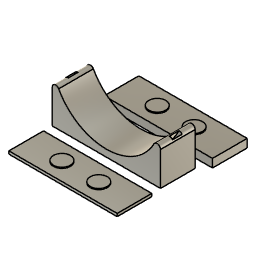
spacer_bandsaw_dust_extraction (Autodesk Fusion 360 design; units mm, degrees)
Autodesk Fusion 360 part; units mm, degrees
sketch "Sketch1" plane through (0, 0, 0) normal (0, 1, 0) x (1, 0, 0)
  circle A0 centre (0, 0) radius 31.25
  line L0 (-31.25, 0) -> (-31.25, 35.25)
  line L1 (-31.25, 35.25) -> (31.25, 35.25)
  line L2 (31.25, 35.25) -> (31.25, 0)
  line L3 (-21.25, 0) -> (-21.25, 33.5)
  line L4 (21.25, 33.5) -> (21.25, 0)
  circle A1 centre (0, 0) radius 32.25
  circle A2 centre (0, 0) radius 34.25
  line L5 (-21.25, 33.5) -> (-21.25, 35.25)
  line L6 (21.25, 33.5) -> (21.25, 35.25)
  dimension "d1" = 62.5
  dimension "d2" = 35.25
  dimension "d3" = 62.5
  dimension "d4" = 10
  dimension "d5" = 10
  dimension "d25" = 1
  dimension "d26" = 3
  constraint coincident A0.centre A1.centre
  constraint coincident A0 L0.start
  constraint tangent A0 L0
  constraint vertical L0
  constraint perpendicular L0 L1
  constraint coincident A0 L2.end
  constraint tangent A0 L2
  constraint coincident L1 L5.end
  constraint perpendicular L1 L5
  constraint coincident L1 L6.end
  constraint perpendicular L1 L6
  measures "d1" diameter of A0
  measures "d2" distance of L0.start L0.end
  measures "d3" distance of L0.end L1.end
extrude "Extrude1" add sketch "Sketch1" along normal blind 20 contours A0 L0 L3 A1 | A0 L2 L4 A1 | A0 L3 L4 A1 | L0 L3 A1 A2 | L2 L4 A1 A2 | L3 L4 A1 A2 | L0 L1 L3 A2 L5 | L1 L2 L4 A2 L6 | L1 L3 L4 A2 L5 L6 makes body 1
fillet "Fillet1" radius 2 2 edges at (-31.25, 10, 0) (31.25, 10, 0) on bodies 1
sketch "Sketch2" plane through (0, 0, -35.25) normal (0, 0, -1) x (1, 0, 0)
  line L0 (31.25, 0) -> (-31.25, 0)
  line L1 (-31.25, -20) -> (31.25, -20)
  line L2 (0, 0) -> (0, -20) construction
  line L3 (-21.25, -10) -> (0, -10) construction
  circle A0 centre (-10.625, -10) radius 5
  circle A1 centre (-10.625, -10) radius 4.9
  circle A2 centre (10.625, -10) radius 5
  circle A3 centre (10.625, -10) radius 4.9
  line L4 (21.25, -10) -> (0, -10) construction
  circle A4 centre (0, -10) radius 3.25
  line L5 (-31.25, 0) -> (-31.25, -20)
  line L6 (31.25, -20) -> (31.25, 0)
  dimension "d10" = 10
  dimension "d14" = -0.1
  dimension "d22" = 6.5
  constraint coincident L2.start origin
  constraint midpoint L1 L2.end
  constraint midpoint L2 L3.end
  constraint midpoint L3 A0.centre
  constraint symmetric L2 L3.start L4.start
  constraint symmetric L2 L3.end L4.end
  constraint symmetric L2 A0 A2
  constraint symmetric L2 A1 A3
  constraint coincident L3.end L4.end
  measures "d10" diameter of A0
  measures "d22" diameter of A4
extrude "Extrude2" cut sketch "Sketch2" against normal blind 1 contours A0 | A1 | A2 | A3 bodies 1
extrude "Extrude3" add sketch "Sketch2" against normal blind 0.6 separate body contours A1 | A3 makes body 2 at (-7.3948, 10.4869, -35.25) makes body 3 at (10.0283, 8.4796, -35.25)
extrude "Extrude4" add sketch "Sketch2" along normal blind 1.6 separate body contours L0 L1 L5 L6 | A0 | A1 | A2 | A3 | A4 makes body 4
extrude "Extrude5" cut sketch "Sketch2" against normal blind 1 from surface at 1.6 contours A0 | A1 | A2 | A3 bodies 4
combine "Combine1" operation add target body 4 tool bodies 2 3
ref_plane "WorkPlane1" through (0, 10, -17.625) normal (0, 1, 0) x (1, 0, 0)
extrude "Extrude6" cut sketch "Sketch1" along normal mid plane 5.5 from surface at 10 contours L0 L3 A1 A2 | L2 L4 A1 A2 | L3 L4 A1 A2 bodies 1
copy_body "CopyPasteBodies1" bodies 4 makes body 5
move_body "Move1" bodies 5 to x (1, 0, 0) y (0, 1, 0) z (0, 0, 1) at (0, 30, 0)
extrude "Extrude7" add 2 faces at (12.3324, 38.3751, -35.85) (-10.7578, 41.5515, -35.85) along direction (0, 0, -1) up to surface end surface through (0, 30, -36.85) normal (0, 0, -1) offset 0 on bodies 5 bodies 5
extrude "Extrude8" add 1 faces at (-10.4167, 36.6667, -36.85) along direction (0, 0, -1) blind 3.2 on bodies 5 bodies 5
move_body "Move2" bodies 4 to x (1, 0, 0) y (0, 1, 0) z (0, 0, 1) at (0, -25, 0)
equation "d2 = 31.25 mm + 4 mm"
equation "d5 = d4"
equation "d32 = ( 1.6 * 2 ) * 1 mm"
